Autodesk Fusion 360 part; units mm, degrees
(part 9 of 25)
  arc A995 (66.6606, 9.2438) -> (66.5391, 8.9505) centre (66.5999, 9.0972) ccw
  line L140 (79.2435, 6.4262) -> (79.2526, 6.4041)
  line L141 (68.5458, 9.1821) -> (70.8777, 6.8502)
  arc A996 (79.3901, 6.4869) -> (79.0968, 6.3655) centre (79.2435, 6.4262) ccw
  line L142 (75.7433, 6.4041) -> (75.7524, 6.4262)
  line L143 (82.2457, 6.4041) -> (82.5144, 7.053)
  arc A997 (74.5979, 9.0106) -> (74.5979, 9.3281) centre (74.5979, 9.1694) ccw
  line L144 (75.7524, 6.4262) -> (79.2435, 6.4262)
  line L145 (73.2468, 8.9006) -> (72.7502, 8.4041)
  arc A998 (73.8956, 9.3281) -> (73.8956, 9.0106) centre (73.8956, 9.1694) ccw
  line L146 (66.2472, 9.4498) -> (66.5998, 9.0972)
  arc A999 (66.4876, 8.9849) -> (66.7121, 9.2094) centre (66.5999, 9.0972) ccw
  line L147 (72.7411, 8.382) -> (72.1118, 8.382)
  arc A1000 (67.0606, 11.5724) -> (67.0606, 11.2549) centre (67.0606, 11.4137) ccw
  arc A1001 (75.631, 8.2918) -> (75.8555, 8.5163) centre (75.7433, 8.4041) ccw
  line L148 (66.2472, 10.8702) -> (66.0563, 10.4094)
  line L149 (72.1118, 8.382) -> (69.5048, 10.989)
  arc A1002 (67.5594, 11.2549) -> (67.5594, 11.5724) centre (67.5594, 11.4137) ccw
  arc A1003 (79.8099, 6.0542) -> (79.6884, 5.7609) centre (79.7492, 5.9076) ccw
  arc A1004 (72.6379, 8.5163) -> (72.8624, 8.2918) centre (72.7501, 8.4041) ccw
  line L150 (81.7491, 5.9076) -> (82.2457, 6.4041)
  arc A1005 (71.0405, 6.4628) -> (71.2651, 6.6873) centre (71.1528, 6.5751) ccw
  line L151 (79.7492, 5.9076) -> (80.398, 5.6388)
  arc A1006 (72.6035, 6.3434) -> (72.8969, 6.4649) centre (72.7502, 6.4042) ccw
  arc A1007 (81.1003, 5.4801) -> (81.1003, 5.7976) centre (81.1003, 5.6389) ccw
  arc A1008 (70.99, 6.9624) -> (70.7655, 6.7379) centre (70.8778, 6.8501) ccw
  arc A1009 (68.5458, 9.0234) -> (68.5458, 9.3408) centre (68.5458, 9.1821) ccw
  arc A1010 (75.8555, 6.2919) -> (75.631, 6.5164) centre (75.7433, 6.4041) ccw
  arc A1011 (67.4986, 9.053) -> (67.6201, 8.7596) centre (67.5593, 8.9063) ccw
  line L152 (80.398, 5.6388) -> (81.1003, 5.6388)
  line L153 (70.8777, 6.8502) -> (71.1528, 6.5751)
  arc A1012 (79.6369, 5.7953) -> (79.8614, 6.0198) centre (79.7491, 5.9076) ccw
  arc A1013 (71.2136, 6.7217) -> (71.0921, 6.4284) centre (71.1529, 6.5751) ccw
  line L154 (68.1051, 9.1821) -> (68.5458, 9.1821)
  line L155 (68.0202, 9.0972) -> (68.1051, 9.1821)
  line L156 (72.7411, 6.4262) -> (72.7502, 6.4041)
  line L157 (81.1003, 5.6388) -> (81.7491, 5.9076)
  line L158 (71.1528, 6.5751) -> (71.5122, 6.4262)
  arc A1014 (81.0395, 5.7855) -> (81.161, 5.4921) centre (81.1003, 5.6388) ccw
  line L159 (1.1279, 35.1317) -> (0.9017, 34.5856)
  arc A1015 (74.5371, 5.7855) -> (74.6586, 5.4921) centre (74.5978, 5.6388) ccw
  arc A1016 (60.0182, 19.5923) -> (59.7936, 19.8168) centre (59.9059, 19.7046) ccw
  arc A1017 (59.7936, 20.8232) -> (60.0182, 21.0477) centre (59.9059, 20.9355) ccw
  line L160 (0.9017, 34.5856) -> (0.9017, 33.9944)
  arc A1018 (1.0605, 34.5856) -> (0.7429, 34.5856) centre (0.9017, 34.5856) ccw
  line L161 (0.9017, 33.9944) -> (1.1279, 33.4483)
  arc A1019 (68.658, 9.2944) -> (68.4335, 9.0698) centre (68.5457, 9.1821) ccw
  line L162 (74.5979, 5.6388) -> (75.2467, 5.9076)
  arc A1020 (72.8624, 6.5164) -> (72.6379, 6.2919) centre (72.7501, 6.4041) ccw
  arc A1021 (68.0809, 8.9505) -> (67.9594, 9.2438) centre (68.0202, 9.0972) ccw
  arc A1022 (73.1345, 5.7953) -> (73.359, 6.0198) centre (73.2468, 5.9076) ccw
  arc A1023 (72.8877, 6.4869) -> (72.5944, 6.3655) centre (72.7411, 6.4262) ccw
  arc A1024 (68.2174, 9.0698) -> (67.9928, 9.2944) centre (68.1051, 9.1821) ccw
  line L163 (73.2468, 5.9076) -> (73.8956, 5.6388)
  arc A1025 (70.7655, 6.7379) -> (70.99, 6.9624) centre (70.8778, 6.8502) ccw
  line L164 (75.2467, 5.9076) -> (75.7433, 6.4041)
  arc A1026 (75.8991, 6.3655) -> (75.6058, 6.4869) centre (75.7525, 6.4262) ccw
  arc A1027 (82.3579, 6.2919) -> (82.1334, 6.5164) centre (82.2456, 6.4041) ccw
  line L165 (79.2526, 6.4041) -> (79.7492, 5.9076)
  arc A1028 (79.3648, 6.5164) -> (79.1403, 6.2919) centre (79.2525, 6.4042) ccw
  arc A1029 (71.5122, 6.585) -> (71.5122, 6.2675) centre (71.5122, 6.4263) ccw
  arc A1030 (80.398, 5.7976) -> (80.398, 5.4801) centre (80.398, 5.6389) ccw
  arc A1031 (81.8099, 5.7609) -> (81.6883, 6.0542) centre (81.7491, 5.9076) ccw
  line L166 (72.7502, 6.4041) -> (73.2468, 5.9076)
  arc A1032 (83.8136, 11.3225) -> (83.4961, 11.3225) centre (83.6548, 11.3225) ccw
  line L167 (73.8956, 5.6388) -> (74.5979, 5.6388)
  arc A1033 (75.5966, 6.4649) -> (75.89, 6.3434) centre (75.7433, 6.4041) ccw
  arc A1034 (73.8348, 5.4921) -> (73.9563, 5.7855) centre (73.8956, 5.6388) ccw
  arc A1035 (1.2746, 35.0709) -> (0.9812, 35.1924) centre (1.1279, 35.1316) ccw
  line L168 (71.5122, 6.4262) -> (72.7411, 6.4262)
  line L169 (82.5144, 7.053) -> (82.5144, 7.7552)
  arc A1036 (75.7524, 6.585) -> (75.7524, 6.2675) centre (75.7524, 6.4263) ccw
  arc A1037 (73.3075, 6.0542) -> (73.186, 5.7609) centre (73.2468, 5.9076) ccw
  arc A1038 (0.7429, 33.9944) -> (1.0605, 33.9944) centre (0.9017, 33.9944) ccw
  arc A1039 (82.6611, 6.9922) -> (82.3678, 7.1137) centre (82.5145, 7.053) ccw
  arc A1040 (71.4515, 6.2795) -> (71.573, 6.5729) centre (71.5122, 6.4262) ccw
  arc A1041 (73.8956, 5.7976) -> (73.8956, 5.4801) centre (73.8956, 5.6389) ccw
  arc A1042 (75.1344, 6.0198) -> (75.359, 5.7953) centre (75.2467, 5.9075) ccw
  arc A1043 (79.1059, 6.3434) -> (79.3993, 6.4649) centre (79.2526, 6.4041) ccw
  arc A1044 (68.1051, 9.3408) -> (68.1051, 9.0234) centre (68.1051, 9.1821) ccw
  arc A1045 (6.6867, 33.177) -> (6.5652, 32.8836) centre (6.626, 33.0303) ccw
  arc A1046 (84.2752, 11.7183) -> (84.0506, 11.9428) centre (84.1629, 11.8305) ccw
  arc A1047 (57.0464, 19.8168) -> (56.8218, 19.5923) centre (56.9341, 19.7046) ccw
  arc A1048 (57.6923, 18.7218) -> (57.9168, 18.9464) centre (57.8045, 18.8341) ccw
  line L170 (83.2309, 8.5029) -> (83.506, 8.778)
  arc A1049 (82.652, 7.8381) -> (82.3586, 7.7165) centre (82.5053, 7.7773) ccw
  arc A1050 (60.0646, 20.9355) -> (59.7471, 20.9355) centre (59.9059, 20.9355) ccw
  line L171 (57.8045, 21.8059) -> (56.9341, 20.9355)
  line L172 (4.004, 35.7759) -> (2.092, 35.7759)
  line L173 (82.5053, 7.7773) -> (83.2309, 8.5029)
  arc A1051 (59.1477, 21.9182) -> (58.9232, 21.6936) centre (59.0355, 21.8059) ccw
  arc A1052 (1.0484, 34.0552) -> (0.755, 33.9337) centre (0.9017, 33.9945) ccw
  arc A1053 (82.3557, 7.053) -> (82.6732, 7.053) centre (82.5145, 7.053) ccw
  line L174 (83.506, 8.778) -> (83.6549, 9.1374)
  arc A1054 (57.8045, 21.9646) -> (57.8045, 21.6471) centre (57.8045, 21.8059) ccw
  arc A1055 (83.3432, 8.3907) -> (83.1187, 8.6152) centre (83.231, 8.5029) ccw
  arc A1056 (59.0355, 18.6753) -> (59.0355, 18.9929) centre (59.0355, 18.8341) ccw
  arc A1057 (57.0928, 20.9355) -> (56.7754, 20.9355) centre (56.9341, 20.9355) ccw
  line L175 (82.5144, 7.7552) -> (82.5053, 7.7773)
  arc A1058 (1.6582, 35.4374) -> (1.4336, 35.6619) centre (1.5459, 35.5496) ccw
  arc A1059 (2.092, 35.9346) -> (2.092, 35.6171) centre (2.092, 35.7759) ccw
  arc A1060 (1.0157, 35.2439) -> (1.2402, 35.0194) centre (1.1279, 35.1317) ccw
  arc A1061 (0.9812, 33.3876) -> (1.2746, 33.5091) centre (1.1279, 33.4484) ccw
  arc A1062 (83.3594, 8.8388) -> (83.6527, 8.7173) centre (83.5061, 8.7781) ccw
  line L176 (59.0355, 18.8341) -> (59.9059, 19.7045)
  arc A1063 (0.755, 34.6463) -> (1.0484, 34.5248) centre (0.9017, 34.5855) ccw
  arc A1064 (83.5426, 11.4348) -> (83.7672, 11.2103) centre (83.6549, 11.3225) ccw
  line L177 (83.6549, 9.1374) -> (83.6549, 11.3225)
  arc A1065 (83.4961, 9.1374) -> (83.8136, 9.1374) centre (83.6548, 9.1374) ccw
  arc A1066 (57.8045, 18.9929) -> (57.8045, 18.6753) centre (57.8045, 18.8341) ccw
  arc A1067 (82.099, 6.4649) -> (82.3924, 6.3434) centre (82.2457, 6.4042) ccw
  arc A1068 (82.393, 7.8896) -> (82.6175, 7.665) centre (82.5053, 7.7773) ccw
  arc A1069 (4.004, 35.6171) -> (4.004, 35.9346) centre (4.004, 35.7759) ccw
  arc A1070 (1.4852, 35.6963) -> (1.6067, 35.403) centre (1.5459, 35.5496) ccw
  arc A1071 (83.1187, 8.6152) -> (83.3432, 8.3907) centre (83.231, 8.503) ccw
  line L178 (2.092, 35.7759) -> (1.5459, 35.5497)
  arc A1072 (58.9232, 18.9464) -> (59.1477, 18.7218) centre (59.0355, 18.8341) ccw
  arc A1073 (82.3678, 7.6945) -> (82.6611, 7.816) centre (82.5145, 7.7553) ccw
  line L179 (59.9059, 19.7045) -> (59.9059, 20.9355)
  line L180 (59.0355, 21.8059) -> (57.8045, 21.8059)
  line L181 (56.9341, 20.9355) -> (56.9341, 19.7045)
  arc A1074 (2.1528, 35.6292) -> (2.0313, 35.9226) centre (2.092, 35.7759) ccw
  arc A1075 (57.9168, 21.6936) -> (57.6923, 21.9182) centre (57.8046, 21.8059) ccw
  arc A1076 (56.8218, 21.0477) -> (57.0464, 20.8232) centre (56.9341, 20.9354) ccw
  line L182 (56.9341, 19.7045) -> (57.8045, 18.8341)
  line L183 (1.5459, 35.5497) -> (1.1279, 35.1317)
  line L184 (59.9059, 20.9355) -> (59.0355, 21.8059)
  arc A1077 (17.4808, 44.6377) -> (17.7053, 44.8622) centre (17.593, 44.7499) ccw
  arc A1078 (56.7754, 19.7045) -> (57.0928, 19.7045) centre (56.9341, 19.7045) ccw
  arc A1079 (83.6183, 8.6658) -> (83.3938, 8.8903) centre (83.5061, 8.7781) ccw
  arc A1080 (83.8016, 9.0767) -> (83.5082, 9.1982) centre (83.6549, 9.1374) ccw
  arc A1081 (59.0355, 21.6471) -> (59.0355, 21.9646) centre (59.0355, 21.8059) ccw
  arc A1082 (59.7471, 19.7045) -> (60.0646, 19.7045) centre (59.9059, 19.7045) ccw
  arc A1083 (17.8886, 31.7487) -> (17.5952, 31.8702) centre (17.7419, 31.8095) ccw
  line L185 (4.5501, 33.0303) -> (4.8319, 33.3121)
  arc A1084 (82.6732, 7.7552) -> (82.3557, 7.7552) centre (82.5145, 7.7552) ccw
  arc A1085 (3.9432, 32.9508) -> (4.0647, 32.6574) centre (4.004, 32.8041) ccw
  line L186 (83.6549, 11.3225) -> (84.1629, 11.8305)
  line L187 (57.8045, 18.8341) -> (59.0355, 18.8341)
  line L188 (2.092, 32.8041) -> (4.004, 32.8041)
  arc A1086 (12.5878, 29.7976) -> (12.4663, 29.5043) centre (12.5271, 29.651) ccw
  arc A1087 (4.4378, 33.1426) -> (4.6623, 32.9181) centre (4.55, 33.0304) ccw
  arc A1088 (15.8547, 29.5043) -> (15.7332, 29.7976) centre (15.7939, 29.651) ccw
  arc A1089 (15.3738, 29.6488) -> (15.4953, 29.3554) centre (15.4345, 29.5021) ccw
  arc A1090 (4.6108, 32.8836) -> (4.4893, 33.177) centre (4.5501, 33.0303) ccw
  line L189 (17.593, 31.4501) -> (17.7419, 31.8095)
  arc A1091 (9.0232, 32.9508) -> (9.1447, 32.6574) centre (9.084, 32.8041) ccw
  arc A1092 (15.6817, 29.7632) -> (15.9062, 29.5387) centre (15.794, 29.651) ccw
  line L190 (12.8865, 29.5021) -> (15.4345, 29.5021)
  arc A1093 (9.084, 32.6454) -> (9.084, 32.9628) centre (9.084, 32.8041) ccw
  line L191 (12.5271, 29.651) -> (12.8865, 29.5021)
  arc A1094 (17.5831, 31.8095) -> (17.9006, 31.8095) centre (17.7419, 31.8095) ccw
  arc A1095 (17.4464, 31.5108) -> (17.7397, 31.3893) centre (17.5931, 31.4501) ccw
  line L192 (17.3179, 45.025) -> (15.1096, 47.2333)
  arc A1096 (6.3441, 33.1534) -> (6.3441, 33.4708) centre (6.3441, 33.3121) ccw
  arc A1097 (9.3498, 32.7424) -> (9.2283, 33.0357) centre (9.2891, 32.8891) ccw
  line L193 (1.1279, 33.4483) -> (1.5459, 33.0303)
  arc A1098 (6.5136, 32.9181) -> (6.7382, 33.1426) centre (6.6259, 33.0304) ccw
  arc A1099 (15.2219, 47.3456) -> (14.9974, 47.1211) centre (15.1097, 47.2334) ccw
  line L194 (15.1096, 47.2333) -> (15.24, 47.3637)
  arc A1100 (17.7397, 44.8107) -> (17.4464, 44.6892) centre (17.5931, 44.7499) ccw
  line L195 (17.593, 44.7499) -> (17.3179, 45.025)
  arc A1101 (19.9142, 47.1562) -> (19.77, 47.4391) centre (19.8421, 47.2977) ccw
  arc A1102 (17.4302, 45.1373) -> (17.2057, 44.9128) centre (17.318, 45.025) ccw
  line L196 (1.5459, 33.0303) -> (2.092, 32.8041)
  arc A1103 (20.1279, 47.309) -> (19.9412, 47.5659) centre (20.0346, 47.4375) ccw
  line L197 (17.7419, 31.8095) -> (17.7419, 44.3905)
  arc A1104 (1.6067, 33.177) -> (1.4852, 32.8836) centre (1.546, 33.0303) ccw
  arc A1105 (4.004, 32.6454) -> (4.004, 32.9628) centre (4.004, 32.8041) ccw
  line L198 (9.084, 32.8041) -> (9.289, 32.889)
  arc A1106 (7.172, 32.9628) -> (7.172, 32.6454) centre (7.172, 32.8041) ccw
  arc A1107 (4.9441, 33.1998) -> (4.7196, 33.4244) centre (4.8319, 33.3121) ccw
  line L199 (4.8319, 33.3121) -> (6.3441, 33.3121)
  arc A1108 (17.2057, 44.9128) -> (17.4302, 45.1373) centre (17.3179, 45.0251) ccw
  arc A1109 (1.2402, 33.5606) -> (1.0157, 33.336) centre (1.128, 33.4483) ccw
  arc A1110 (15.3523, 47.2514) -> (15.1277, 47.4759) centre (15.24, 47.3636) ccw
  arc A1111 (12.8257, 29.3554) -> (12.9472, 29.6488) centre (12.8865, 29.5021) ccw
  line L200 (17.7419, 44.3905) -> (17.593, 44.7499)
  line L201 (6.3441, 33.3121) -> (6.6259, 33.0303)
  arc A1112 (12.8865, 29.6609) -> (12.8865, 29.3434) centre (12.8865, 29.5022) ccw
  line L202 (15.24, 47.3637) -> (15.51, 47.0937)
  arc A1113 (9.4013, 33.0013) -> (9.1768, 32.7768) centre (9.2891, 32.8891) ccw
  line L203 (7.172, 32.8041) -> (9.084, 32.8041)
  arc A1114 (7.1113, 32.6574) -> (7.2328, 32.9508) centre (7.1721, 32.8041) ccw
  arc A1115 (15.4345, 29.3434) -> (15.4345, 29.6609) centre (15.4345, 29.5022) ccw
  arc A1116 (6.4564, 33.4244) -> (6.2319, 33.1998) centre (6.3442, 33.3121) ccw
  arc A1117 (1.4336, 32.9181) -> (1.6582, 33.1426) centre (1.5459, 33.0304) ccw
  arc A1118 (12.4148, 29.5387) -> (12.6393, 29.7632) centre (12.5271, 29.651) ccw
  arc A1119 (17.7053, 31.3378) -> (17.4808, 31.5623) centre (17.593, 31.4501) ccw
  line L204 (15.4345, 29.5021) -> (15.7939, 29.651)
  line L205 (4.004, 32.8041) -> (4.5501, 33.0303)
  line L206 (6.6259, 33.0303) -> (7.172, 32.8041)
  arc A1120 (2.0313, 32.6574) -> (2.1528, 32.9508) centre (2.0921, 32.8041) ccw
  arc A1121 (4.8319, 33.4708) -> (4.8319, 33.1534) centre (4.8319, 33.3121) ccw
  arc A1122 (2.092, 32.9628) -> (2.092, 32.6454) centre (2.092, 32.8041) ccw
  line L207 (15.7939, 29.651) -> (17.593, 31.4501)
  arc A1123 (17.9006, 44.3905) -> (17.5831, 44.3905) centre (17.7419, 44.3905) ccw
  arc A1124 (17.5952, 44.3298) -> (17.8886, 44.4513) centre (17.7419, 44.3905) ccw
  arc A1125 (14.9974, 47.3456) -> (15.2219, 47.1211) centre (15.1097, 47.2334) ccw
  line L208 (9.289, 32.889) -> (12.5271, 29.651)
  arc A1126 (20.2526, 47.431) -> (20.0281, 47.6555) centre (20.1403, 47.5433) ccw
  arc A1127 (21.1781, 46.6782) -> (21.2996, 46.9716) centre (21.2388, 46.8249) ccw
  line L209 (19.4039, 47.1161) -> (19.6301, 47.1896)
  arc A1128 (16.8611, 46.6662) -> (16.8611, 46.9836) centre (16.8611, 46.8249) ccw
  arc A1129 (18.0719, 47.6555) -> (17.8473, 47.431) centre (17.9596, 47.5433) ccw
  arc A1130 (18.9062, 46.9221) -> (18.9559, 47.2357) centre (18.9311, 47.0789) ccw
  arc A1131 (19.05, 49.3712) -> (19.05, 49.6887) centre (19.05, 49.53) ccw
  arc A1132 (19.2088, 49.53) -> (18.8913, 49.53) centre (19.0501, 49.53) ccw
  line L210 (20.1404, 47.5433) -> (20.59, 47.0937)
  line L211 (19.05, 47.0789) -> (19.05, 49.53)
  line L212 (16.1589, 46.8249) -> (16.8611, 46.8249)
  line L213 (19.05, 49.53) -> (19.05, 47.0789)
  arc A1133 (18.5189, 47.3406) -> (18.4208, 47.0386) centre (18.4699, 47.1896) ccw
  arc A1134 (18.33, 47.4391) -> (18.1858, 47.1562) centre (18.2579, 47.2977) ccw
  arc A1135 (19.5581, 47.3311) -> (19.7022, 47.0482) centre (19.6302, 47.1897) ccw
  line L214 (18.2579, 47.2976) -> (18.4699, 47.1896)
  arc A1136 (17.9532, 47.3252) -> (18.1777, 47.5497) centre (18.0655, 47.4375) ccw
  line L215 (19.05, 47.0789) -> (19.1689, 47.0789)
  line L216 (17.9596, 47.5433) -> (18.0655, 47.4374)
  line L217 (17.51, 47.0937) -> (17.9596, 47.5433)
  line L218 (15.51, 47.0937) -> (16.1589, 46.8249)
  arc A1137 (19.1441, 47.2357) -> (19.1938, 46.9221) centre (19.169, 47.0789) ccw
  arc A1138 (17.3977, 47.2059) -> (17.6222, 46.9814) centre (17.5099, 47.0936) ccw
  arc A1139 (19.7488, 47.426) -> (19.9354, 47.1692) centre (19.8421, 47.2976) ccw
  line L219 (20.0345, 47.4374) -> (20.1404, 47.5433)
  line L220 (19.6301, 47.1896) -> (19.8421, 47.2976)
  arc A1140 (16.1589, 46.9836) -> (16.1589, 46.6662) centre (16.1589, 46.8249) ccw
  line L221 (18.4699, 47.1896) -> (18.6961, 47.1161)
  arc A1141 (15.3523, 47.4759) -> (15.1277, 47.2514) centre (15.24, 47.3636) ccw
  line L222 (18.6961, 47.1161) -> (18.9311, 47.0789)
  arc A1142 (18.7209, 47.2729) -> (18.6713, 46.9593) centre (18.6961, 47.1161) ccw
  line L223 (19.8421, 47.2976) -> (20.0345, 47.4374)
  line L224 (18.9311, 47.0789) -> (19.05, 47.0789)
  arc A1143 (19.1689, 46.9202) -> (19.1689, 47.2377) centre (19.1689, 47.0789) ccw
  arc A1144 (18.8912, 47.0789) -> (19.2087, 47.0789) centre (19.05, 47.0789) ccw
  arc A1145 (19.6792, 47.0386) -> (19.5811, 47.3406) centre (19.6302, 47.1896) ccw
  line L225 (20.59, 47.0937) -> (21.2389, 46.8249)
  arc A1146 (18.1646, 47.1692) -> (18.3512, 47.426) centre (18.2579, 47.2976) ccw
  arc A1147 (18.3978, 47.0482) -> (18.5419, 47.3311) centre (18.4699, 47.1897) ccw
  arc A1148 (15.5708, 47.2403) -> (15.4493, 46.947) centre (15.51, 47.0936) ccw
  line L226 (16.8611, 46.8249) -> (17.51, 47.0937)
  arc A1149 (19.4287, 46.9593) -> (19.3791, 47.2729) centre (19.4039, 47.1161) ccw
  arc A1150 (18.8913, 47.0789) -> (19.2088, 47.0789) centre (19.0501, 47.0789) ccw
  arc A1151 (19.05, 49.6887) -> (19.05, 49.3712) centre (19.05, 49.53) ccw
  arc A1152 (19.05, 47.2377) -> (19.05, 46.9202) centre (19.05, 47.0789) ccw
  line L227 (18.0655, 47.4374) -> (18.2579, 47.2976)
  line L228 (19.1689, 47.0789) -> (19.4039, 47.1161)
  arc A1153 (17.5707, 46.947) -> (17.4492, 47.2403) centre (17.5099, 47.0936) ccw
  arc A1154 (19.05, 46.9202) -> (19.05, 47.2377) centre (19.05, 47.0789) ccw
  arc A1155 (16.8004, 46.9716) -> (16.9219, 46.6782) centre (16.8611, 46.8249) ccw
  arc A1156 (19.9223, 47.5497) -> (20.1468, 47.3252) centre (20.0346, 47.4375) ccw
  arc A1157 (15.3978, 46.9814) -> (15.6223, 47.2059) centre (15.51, 47.0936) ccw
  arc A1158 (18.0719, 47.431) -> (17.8473, 47.6555) centre (17.9596, 47.5433) ccw
  arc A1159 (19.3548, 47.2671) -> (19.453, 46.9651) centre (19.4039, 47.1161) ccw
  arc A1160 (18.1588, 47.5659) -> (17.9721, 47.309) centre (18.0654, 47.4375) ccw
  arc A1161 (20.2526, 47.6555) -> (20.0281, 47.431) centre (20.1403, 47.5433) ccw
  arc A1162 (20.4778, 46.9814) -> (20.7023, 47.2059) centre (20.59, 47.0936) ccw
  arc A1163 (20.6508, 47.2403) -> (20.5293, 46.947) centre (20.59, 47.0936) ccw
  arc A1164 (18.9311, 47.2377) -> (18.9311, 46.9202) centre (18.9311, 47.0789) ccw
  arc A1165 (16.0981, 46.6782) -> (16.2196, 46.9716) centre (16.1589, 46.8249) ccw
  arc A1166 (18.647, 46.9651) -> (18.7452, 47.2671) centre (18.6961, 47.1161) ccw
  arc A1167 (27.0488, 48.5057) -> (26.8621, 48.2488) centre (26.9554, 48.3773) ccw
  arc A1168 (25.6904, 47.9114) -> (25.8119, 47.618) centre (25.7511, 47.7647) ccw
  arc A1169 (22.6507, 46.947) -> (22.5292, 47.2403) centre (22.59, 47.0936) ccw
  line L229 (24.4, 48.0335) -> (25.0489, 47.7647)
  arc A1170 (21.8804, 46.9716) -> (22.0019, 46.6782) centre (21.9411, 46.8249) ccw
  arc A1171 (27.7962, 47.8619) -> (27.8459, 48.1755) centre (27.8211, 48.0187) ccw
  arc A1172 (24.9881, 47.618) -> (25.1096, 47.9114) centre (25.0489, 47.7647) ccw
  arc A1173 (24.1587, 48.4993) -> (23.9342, 48.2747) centre (24.0465, 48.387) ccw
  arc A1174 (28.3187, 47.8991) -> (28.2691, 48.2127) centre (28.2939, 48.0559) ccw
  arc A1175 (23.1965, 48.2391) -> (23.514, 48.2391) centre (23.3553, 48.2391) ccw
  arc A1176 (28.0589, 47.86) -> (28.0589, 48.1775) centre (28.0589, 48.0187) ccw
  arc A1177 (27.8211, 48.1774) -> (27.8211, 47.86) centre (27.8211, 48.0187) ccw
  arc A1178 (25.7511, 47.606) -> (25.7511, 47.9235) centre (25.7511, 47.7648) ccw
  arc A1179 (26.9619, 48.5953) -> (26.7373, 48.3708) centre (26.8496, 48.4831) ccw
  arc A1180 (26.4607, 47.8868) -> (26.3392, 48.1801) centre (26.3999, 48.0335) ccw
  arc A1181 (24.2878, 47.9212) -> (24.5123, 48.1457) centre (24.4001, 48.0335) ccw
  arc A1182 (27.0546, 48.109) -> (27.2412, 48.3658) centre (27.1479, 48.2374) ccw
  arc A1183 (23.1988, 47.478) -> (22.9743, 47.7025) centre (23.0866, 47.5903) ccw
  line L230 (26.4, 48.0335) -> (26.8496, 48.4831)
  line L231 (27.1479, 48.2374) -> (27.3599, 48.1294)
  arc A1184 (27.22, 48.3789) -> (27.0758, 48.096) centre (27.1479, 48.2374) ccw
  arc A1185 (27.94, 48.1775) -> (27.94, 47.86) centre (27.94, 48.0187) ccw
  arc A1186 (21.2389, 46.9836) -> (21.2389, 46.6662) centre (21.2389, 46.8249) ccw
  line L232 (27.3599, 48.1294) -> (27.5861, 48.0559)
  line L233 (25.7511, 47.7647) -> (26.4, 48.0335)
  line L234 (21.2389, 46.8249) -> (21.9411, 46.8249)
  arc A1187 (23.502, 48.1783) -> (23.2086, 48.2998) centre (23.3553, 48.239) ccw
  line L235 (23.3553, 48.387) -> (24.0465, 48.387)
  arc A1188 (27.537, 47.9049) -> (27.6352, 48.2069) centre (27.5861, 48.0559) ccw
  arc A1189 (26.9619, 48.3708) -> (26.7373, 48.5953) centre (26.8496, 48.483) ccw
  arc A1190 (28.0987, 49.53) -> (27.7812, 49.53) centre (27.94, 49.53) ccw
  line L236 (21.9411, 46.8249) -> (22.59, 47.0937)
  arc A1191 (26.2877, 48.1457) -> (26.5122, 47.9212) centre (26.4, 48.0335) ccw
  arc A1192 (27.2878, 47.988) -> (27.4319, 48.2709) centre (27.3599, 48.1294) ccw
  arc A1193 (19.2087, 49.53) -> (18.8912, 49.53) centre (19.05, 49.53) ccw
  arc A1194 (28.0988, 49.53) -> (27.7813, 49.53) centre (27.9401, 49.53) ccw
  arc A1195 (26.8432, 48.265) -> (27.0677, 48.4895) centre (26.9554, 48.3773) ccw
  line L237 (23.0865, 47.5902) -> (23.3553, 48.2391)
  arc A1196 (27.4089, 48.2804) -> (27.3108, 47.9784) centre (27.3599, 48.1294) ccw
  arc A1197 (21.9411, 46.6662) -> (21.9411, 46.9836) centre (21.9411, 46.8249) ccw
  line L238 (27.8211, 48.0187) -> (27.94, 48.0187)
  arc A1198 (25.0489, 47.9235) -> (25.0489, 47.606) centre (25.0489, 47.7648) ccw
  arc A1199 (27.94, 47.8599) -> (27.94, 48.1774) centre (27.94, 48.0187) ccw
  line L239 (22.59, 47.0937) -> (23.0865, 47.5902)
  arc A1200 (24.4608, 48.1801) -> (24.3393, 47.8868) centre (24.4, 48.0335) ccw
  line L240 (27.5861, 48.0559) -> (27.8211, 48.0187)
  line L241 (27.94, 48.0187) -> (28.0589, 48.0187)
  line L242 (28.0589, 48.0187) -> (28.2939, 48.0559)
  line L243 (24.0465, 48.387) -> (24.4, 48.0335)
  arc A1201 (22.9399, 47.651) -> (23.2332, 47.5295) centre (23.0866, 47.5903) ccw
  arc A1202 (27.6109, 48.2127) -> (27.5613, 47.8991) centre (27.5861, 48.0559) ccw
  arc A1203 (27.7813, 48.0187) -> (28.0988, 48.0187) centre (27.9401, 48.0187) ccw
  arc A1204 (24.0465, 48.2283) -> (24.0465, 48.5457) centre (24.0465, 48.387) ccw
  arc A1205 (22.4777, 47.2059) -> (22.7022, 46.9814) centre (22.5899, 47.0936) ccw
  line L244 (25.0489, 47.7647) -> (25.7511, 47.7647)
  arc A1206 (27.94, 49.3712) -> (27.94, 49.6887) centre (27.94, 49.53) ccw
  arc A1207 (23.514, 48.387) -> (23.1965, 48.387) centre (23.3553, 48.387) ccw
  line L245 (26.9555, 48.3772) -> (27.1479, 48.2374)
  arc A1208 (23.3553, 48.5457) -> (23.3553, 48.2283) centre (23.3553, 48.387) ccw
  line L246 (23.3553, 48.2391) -> (23.3553, 48.387)
  line L247 (26.8496, 48.4831) -> (26.9555, 48.3772)
  line L248 (30.48, 49.53) -> (30.48, 48.0187)
  line L249 (30.8339, 48.0559) -> (31.0601, 48.1294)
  arc A1209 (28.6388, 48.3658) -> (28.8254, 48.109) centre (28.7321, 48.2374) ccw
  arc A1210 (30.48, 49.6887) -> (30.48, 49.3712) centre (30.48, 49.53) ccw
  line L250 (29.6879, 48.2374) -> (29.8999, 48.1294)
  arc A1211 (29.3384, 48.8001) -> (29.0816, 48.6135) centre (29.21, 48.7068) ccw
  line L251 (29.21, 48.7068) -> (29.3272, 48.5455)
  arc A1212 (29.3832, 48.265) -> (29.6077, 48.4895) centre (29.4955, 48.3773) ccw
  arc A1213 (29.3384, 48.6135) -> (29.0816, 48.8001) centre (29.21, 48.7068) ccw
  line L252 (29.0928, 48.5455) -> (29.21, 48.7068)
  arc A1214 (27.94, 49.6887) -> (27.94, 49.3712) centre (27.94, 49.53) ccw
  line L253 (31.0601, 48.1294) -> (31.2721, 48.2374)
  arc A1215 (28.2448, 48.2069) -> (28.343, 47.9049) centre (28.2939, 48.0559) ccw
  line L254 (31.2721, 48.2374) -> (31.4645, 48.3772)
  arc A1216 (31.3442, 48.096) -> (31.2, 48.3789) centre (31.2721, 48.2375) ccw
  arc A1217 (30.3212, 48.0187) -> (30.6387, 48.0187) centre (30.48, 48.0187) ccw
  arc A1218 (29.9489, 48.2804) -> (29.8508, 47.9784) centre (29.8999, 48.1294) ccw
  arc A1219 (28.8042, 48.096) -> (28.66, 48.3789) centre (28.7321, 48.2375) ccw
  arc A1220 (30.3213, 48.0187) -> (30.6388, 48.0187) centre (30.4801, 48.0187) ccw
  arc A1221 (29.8278, 47.988) -> (29.9719, 48.2709) centre (29.8999, 48.1294) ccw
  arc A1222 (30.3362, 47.8619) -> (30.3859, 48.1755) centre (30.3611, 48.0187) ccw
  line L255 (30.5989, 48.0187) -> (30.8339, 48.0559)
  arc A1223 (30.8587, 47.8991) -> (30.8091, 48.2127) centre (30.8339, 48.0559) ccw
  arc A1224 (28.5692, 47.9784) -> (28.4711, 48.2804) centre (28.5202, 48.1294) ccw
  arc A1225 (30.48, 47.8599) -> (30.48, 48.1774) centre (30.48, 48.0187) ccw
  line L256 (30.48, 48.0187) -> (30.5989, 48.0187)
  line L257 (28.9245, 48.3772) -> (29.0928, 48.5455)
  arc A1226 (30.3611, 48.1774) -> (30.3611, 47.86) centre (30.3611, 48.0187) ccw
  arc A1227 (29.0179, 48.2488) -> (28.8312, 48.5057) centre (28.9246, 48.3773) ccw
  arc A1228 (30.077, 47.9049) -> (30.1752, 48.2069) centre (30.1261, 48.0559) ccw
  arc A1229 (30.5741, 48.1755) -> (30.6238, 47.8619) centre (30.599, 48.0187) ccw
  line L258 (27.94, 48.0187) -> (27.94, 49.53)
  arc A1230 (28.8123, 48.4895) -> (29.0368, 48.265) centre (28.9246, 48.3773) ccw
  arc A1231 (28.4481, 48.2709) -> (28.5922, 47.988) centre (28.5202, 48.1294) ccw
  arc A1232 (30.1509, 48.2127) -> (30.1013, 47.8991) centre (30.1261, 48.0559) ccw
  arc A1233 (28.9643, 48.6388) -> (29.2212, 48.4521) centre (29.0928, 48.5455) ccw
  arc A1234 (29.5888, 48.5057) -> (29.4021, 48.2488) centre (29.4955, 48.3772) ccw
  line L259 (30.1261, 48.0559) -> (30.3611, 48.0187)
  line L260 (29.3272, 48.5455) -> (29.4955, 48.3772)
  line L261 (31.5704, 48.4831) -> (32.02, 48.0335)
  arc A1235 (30.5989, 47.86) -> (30.5989, 48.1775) centre (30.5989, 48.0187) ccw
  arc A1236 (30.48, 49.3712) -> (30.48, 49.6887) centre (30.48, 49.53) ccw
  line L262 (30.48, 48.0187) -> (30.48, 49.53)
  line L263 (28.2939, 48.0559) -> (28.5201, 48.1294)
  line L264 (31.4645, 48.3772) -> (31.5704, 48.4831)
  line L265 (29.4955, 48.3772) -> (29.6879, 48.2374)
  arc A1237 (31.3523, 48.4895) -> (31.5768, 48.265) centre (31.4645, 48.3773) ccw
  arc A1238 (29.205, 48.4332) -> (28.9805, 48.6577) centre (29.0927, 48.5455) ccw
  line L266 (28.7321, 48.2374) -> (28.9245, 48.3772)
  line L267 (30.3611, 48.0187) -> (30.48, 48.0187)
  arc A1239 (30.7848, 48.2069) -> (30.883, 47.9049) centre (30.8339, 48.0559) ccw
  arc A1240 (29.4395, 48.6577) -> (29.215, 48.4332) centre (29.3272, 48.5455) ccw
  line L268 (28.5201, 48.1294) -> (28.7321, 48.2374)
  arc A1241 (29.76, 48.3789) -> (29.6158, 48.096) centre (29.6879, 48.2374) ccw
  arc A1242 (29.1988, 48.4521) -> (29.4557, 48.6388) centre (29.3273, 48.5455) ccw
  line L269 (29.8999, 48.1294) -> (30.1261, 48.0559)
  arc A1243 (30.6388, 49.53) -> (30.3213, 49.53) centre (30.4801, 49.53) ccw
  arc A1244 (29.5946, 48.109) -> (29.7812, 48.3658) centre (29.6879, 48.2374) ccw
  line L270 (27.94, 49.53) -> (27.94, 48.0187)
  arc A1245 (31.1092, 47.9784) -> (31.0111, 48.2804) centre (31.0602, 48.1294) ccw
  arc A1246 (27.7812, 48.0187) -> (28.0987, 48.0187) centre (27.94, 48.0187) ccw
  line L271 (24.0548, 44.6572) -> (24.5156, 44.4663)
  arc A1247 (30.48, 48.1775) -> (30.48, 47.86) centre (30.48, 48.0187) ccw
  arc A1248 (34.5214, 47.8776) -> (34.6428, 48.171) centre (34.5821, 48.0243) ccw
  arc A1249 (25.5601, 46.8566) -> (25.5601, 46.5391) centre (25.5601, 46.6979) ccw
  arc A1250 (23.8144, 45.1221) -> (23.5899, 44.8976) centre (23.7021, 45.0099) ccw
  arc A1251 (25.4478, 46.5856) -> (25.6724, 46.8102) centre (25.5601, 46.6979) ccw
  line L272 (33.3711, 47.7647) -> (34.02, 48.0335)
  arc A1252 (28.0341, 48.1755) -> (28.0838, 47.8619) centre (28.059, 48.0187) ccw
  arc A1253 (32.6689, 47.9235) -> (32.6689, 47.606) centre (32.6689, 47.7648) ccw
  arc A1254 (33.8849, 46.5391) -> (33.8849, 46.8566) centre (33.8849, 46.6979) ccw
  line L273 (34.29, 48.3035) -> (34.56, 48.0335)
  arc A1255 (31.5579, 48.2488) -> (31.3712, 48.5057) centre (31.4646, 48.3773) ccw
  arc A1256 (34.4023, 48.1912) -> (34.1777, 48.4157) centre (34.29, 48.3035) ccw
  arc A1257 (24.5156, 44.6251) -> (24.5156, 44.3076) centre (24.5156, 44.4664) ccw
  line L274 (33.8849, 46.6979) -> (25.5601, 46.6979)
  arc A1258 (25.0144, 44.3076) -> (25.0144, 44.6251) centre (25.0144, 44.4664) ccw
  line L275 (25.0144, 44.4663) -> (25.4752, 44.6572)
  arc A1259 (23.658, 45.5314) -> (23.3646, 45.4099) centre (23.5113, 45.4706) ccw
  arc A1260 (24.4549, 44.3196) -> (24.5764, 44.613) centre (24.5157, 44.4663) ccw
  line L276 (34.56, 48.0335) -> (34.5821, 48.0243)
  arc A1261 (31.9078, 47.9212) -> (32.1323, 48.1457) centre (32.0201, 48.0335) ccw
  arc A1262 (34.7409, 48.0243) -> (34.4234, 48.0243) centre (34.5822, 48.0243) ccw
  arc A1263 (31.1788, 48.3658) -> (31.3654, 48.109) centre (31.2721, 48.2374) ccw
  line L277 (24.5156, 44.4663) -> (25.0144, 44.4663)
  line L278 (23.7022, 45.0098) -> (24.0548, 44.6572)
  arc A1264 (24.1156, 44.8038) -> (23.9941, 44.5105) centre (24.0549, 44.6572) ccw
  arc A1265 (33.3104, 47.9114) -> (33.4319, 47.618) centre (33.3711, 47.7647) ccw
  line L279 (34.5821, 47.3951) -> (33.8849, 46.6979)
  line L280 (23.7022, 46.4302) -> (23.5113, 45.9694)
  arc A1266 (25.0144, 46.8149) -> (25.0144, 47.1324) centre (25.0144, 46.9737) ccw
  arc A1267 (31.6826, 48.3708) -> (31.4581, 48.5953) centre (31.5704, 48.483) ccw
  arc A1268 (23.6701, 45.9694) -> (23.3526, 45.9694) centre (23.5113, 45.9694) ccw
  line L281 (23.5113, 45.9694) -> (23.5113, 45.4706)
  arc A1269 (33.3711, 47.606) -> (33.3711, 47.9235) centre (33.3711, 47.7648) ccw
  arc A1270 (34.4234, 47.3951) -> (34.7409, 47.3951) centre (34.5822, 47.3951) ccw
  arc A1271 (32.6081, 47.618) -> (32.7296, 47.9114) centre (32.6689, 47.7647) ccw
  arc A1272 (25.4144, 46.6362) -> (25.5359, 46.9295) centre (25.4752, 46.7828) ccw
  line L282 (32.02, 48.0335) -> (32.6689, 47.7647)
  arc A1273 (25.5359, 44.5105) -> (25.4144, 44.8038) centre (25.4752, 44.6572) ccw
  arc A1274 (24.1671, 46.6706) -> (23.9426, 46.8951) centre (24.0549, 46.7829) ccw
  arc A1275 (23.3646, 46.0301) -> (23.658, 45.9086) centre (23.5113, 45.9694) ccw
  line L283 (25.4752, 46.7828) -> (25.0144, 46.9737)
  arc A1276 (23.5555, 44.9491) -> (23.8488, 45.0706) centre (23.7021, 45.0099) ccw
  line L284 (32.6689, 47.7647) -> (33.3711, 47.7647)
  arc A1277 (34.4023, 48.4157) -> (34.1777, 48.1912) centre (34.29, 48.3035) ccw
  arc A1278 (30.9881, 48.2709) -> (31.1322, 47.988) centre (31.0602, 48.1294) ccw
  arc A1279 (30.6387, 49.53) -> (30.3212, 49.53) centre (30.48, 49.53) ccw
  arc A1280 (34.0807, 47.8868) -> (33.9592, 48.1801) centre (34.02, 48.0335) ccw
  arc A1281 (33.7727, 46.8102) -> (33.9972, 46.5856) centre (33.885, 46.6979) ccw
  line L285 (25.0144, 46.9737) -> (24.5156, 46.9737)
  arc A1282 (31.6826, 48.5953) -> (31.4581, 48.3708) centre (31.5704, 48.483) ccw
  line L286 (25.5601, 46.6979) -> (25.4752, 46.7828)
  arc A1283 (33.9077, 48.1457) -> (34.1322, 47.9212) centre (34.02, 48.0335) ccw
  line L287 (24.5156, 46.9737) -> (24.0548, 46.7828)
  line L288 (34.5821, 48.0243) -> (34.5821, 47.3951)
  arc A1284 (23.8488, 46.3694) -> (23.5555, 46.4909) centre (23.7021, 46.4301) ccw
  arc A1285 (34.6208, 48.1801) -> (34.4993, 47.8868) centre (34.56, 48.0335) ccw
  arc A1286 (34.6944, 47.2828) -> (34.4698, 47.5073) centre (34.5821, 47.395) ccw
  arc A1287 (25.5874, 46.8951) -> (25.3629, 46.6706) centre (25.4752, 46.7829) ccw
  arc A1288 (23.9941, 46.9295) -> (24.1156, 46.6362) centre (24.0549, 46.7828) ccw
  arc A1289 (24.9536, 44.613) -> (25.0751, 44.3196) centre (25.0144, 44.4663) ccw
  arc A1290 (24.5156, 47.1324) -> (24.5156, 46.8149) centre (24.5156, 46.9737) ccw
  arc A1291 (29.7976, 42.4032) -> (29.5043, 42.5247) centre (29.651, 42.4639) ccw
  line L289 (35.9156, 33.6167) -> (35.9156, 34.9633)
  arc A1292 (35.7568, 33.6167) -> (36.0743, 33.6167) centre (35.9156, 33.6167) ccw
  arc A1293 (24.5764, 46.827) -> (24.4549, 47.1204) centre (24.5156, 46.9737) ccw
  arc A1294 (29.3554, 42.1653) -> (29.6488, 42.0438) centre (29.5021, 42.1045) ccw
  line L290 (34.02, 48.0335) -> (34.29, 48.3035)
  arc A1295 (32.8567, 35.3802) -> (33.0812, 35.1556) centre (32.9689, 35.2679) ccw
  line L291 (31.5555, 33.3121) -> (32.969, 33.3121)
  arc A1296 (35.8033, 34.8511) -> (36.0279, 35.0756) centre (35.9156, 34.9634) ccw
  line L292 (23.5113, 45.4706) -> (23.7022, 45.0098)
  arc A1297 (31.0838, 33.3487) -> (31.3083, 33.5732) centre (31.196, 33.4609) ccw
  line L293 (29.9261, 42.739) -> (29.651, 42.4639)
  arc A1298 (29.3434, 35.3655) -> (29.6609, 35.3655) centre (29.5022, 35.3655) ccw
  arc A1299 (23.5899, 46.5424) -> (23.8144, 46.3179) centre (23.7021, 46.4301) ccw
  line L294 (34.9633, 35.9156) -> (33.6167, 35.9156)
  arc A1300 (34.9633, 35.7568) -> (34.9633, 36.0743) centre (34.9633, 35.9156) ccw
  arc A1301 (25.5601, 44.9008) -> (25.5601, 44.5834) centre (25.5601, 44.7421) ccw
  line L295 (29.5021, 42.1045) -> (29.5021, 35.3655)
  arc A1302 (29.9261, 34.8897) -> (29.9261, 34.5722) centre (29.9261, 34.7309) ccw
  line L296 (29.651, 42.4639) -> (29.5021, 42.1045)
  arc A1303 (30.8087, 33.6238) -> (31.0332, 33.8483) centre (30.921, 33.7361) ccw
  arc A1304 (30.0383, 42.6268) -> (29.8138, 42.8513) centre (29.9261, 42.7391) ccw
  arc A1305 (25.3629, 44.7694) -> (25.5874, 44.5449) centre (25.4751, 44.6571) ccw
  arc A1306 (23.9426, 44.5449) -> (24.1671, 44.7694) centre (24.0548, 44.6571) ccw
  line L297 (35.9156, 34.9633) -> (34.9633, 35.9156)
  line L298 (30.921, 33.7361) -> (31.1961, 33.461)
  arc A1307 (30.0383, 34.8432) -> (29.8138, 34.6187) centre (29.9261, 34.7309) ccw
  arc A1308 (31.4947, 33.1654) -> (31.6162, 33.4588) centre (31.5555, 33.3121) ccw
  arc A1309 (33.0812, 33.4244) -> (32.8567, 33.1998) centre (32.9689, 33.3121) ccw
  arc A1310 (36.0279, 33.5044) -> (35.8033, 33.7289) centre (35.9156, 33.6167) ccw
  arc A1311 (36.0743, 34.9633) -> (35.7568, 34.9633) centre (35.9156, 34.9633) ccw
  arc A1312 (34.8511, 32.7767) -> (35.0756, 32.5521) centre (34.9634, 32.6644) ccw
  arc A1313 (32.0414, 44.6298) -> (31.8169, 44.8544) centre (31.9292, 44.7421) ccw
  line L299 (29.651, 35.0061) -> (29.9261, 34.731)
  arc A1314 (29.8138, 34.6187) -> (30.0383, 34.8432) centre (29.9261, 34.7309) ccw
  arc A1315 (32.1551, 35.4266) -> (32.1551, 35.1091) centre (32.1551, 35.2678) ccw
  arc A1316 (33.7289, 35.8033) -> (33.5044, 36.0279) centre (33.6167, 35.9156) ccw
  line L300 (31.1961, 33.461) -> (31.5555, 33.3121)
  line L301 (34.9633, 32.6644) -> (35.9156, 33.6167)
  line L302 (29.5021, 35.3655) -> (29.651, 35.0061)
  arc A1317 (29.9261, 42.8978) -> (29.9261, 42.5803) centre (29.9261, 42.739) ccw
  arc A1318 (32.0808, 48.1801) -> (31.9593, 47.8868) centre (32.0201, 48.0335) ccw
  line L303 (24.0548, 46.7828) -> (23.7022, 46.4302)
  arc A1319 (34.4478, 47.9212) -> (34.6723, 48.1457) centre (34.5601, 48.0335) ccw
  arc A1320 (33.6167, 36.0743) -> (33.6167, 35.7568) centre (33.6167, 35.9156) ccw
  arc A1321 (31.5555, 33.4708) -> (31.5555, 33.1534) centre (31.5555, 33.3121) ccw
  arc A1322 (31.0332, 33.8483) -> (30.8087, 33.6238) centre (30.921, 33.7361) ccw
  arc A1323 (33.6167, 32.8231) -> (33.6167, 32.5057) centre (33.6167, 32.6644) ccw
  arc A1324 (29.7632, 35.1183) -> (29.5387, 34.8938) centre (29.651, 35.006) ccw
  arc A1325 (35.0756, 36.0279) -> (34.8511, 35.8033) centre (34.9634, 35.9156) ccw
  arc A1326 (23.3526, 45.4706) -> (23.6701, 45.4706) centre (23.5113, 45.4706) ccw
  arc A1327 (25.6724, 44.6298) -> (25.4478, 44.8544) centre (25.5601, 44.7421) ccw
  line L304 (25.5601, 44.7421) -> (31.9291, 44.7421)
  arc A1328 (25.0751, 47.1204) -> (24.9536, 46.827) centre (25.0144, 46.9737) ccw
  arc A1329 (29.5387, 42.5762) -> (29.7632, 42.3517) centre (29.6509, 42.4639) ccw
  line L305 (33.6167, 35.9156) -> (32.969, 35.2679)
  line L306 (32.969, 35.2679) -> (32.1551, 35.2679)
  arc A1330 (31.9291, 44.5834) -> (31.9291, 44.9008) centre (31.9291, 44.7421) ccw
  arc A1331 (29.5043, 34.9453) -> (29.7976, 35.0668) centre (29.651, 35.0061) ccw
  arc A1332 (29.6609, 42.1045) -> (29.3434, 42.1045) centre (29.5022, 42.1045) ccw
  arc A1333 (29.9261, 42.5803) -> (29.9261, 42.8978) centre (29.9261, 42.739) ccw
  line L307 (56.6547, 44.4709) -> (56.6547, 44.323)
  arc A1334 (58.8319, 46.0318) -> (58.7104, 45.7384) centre (58.7711, 45.8851) ccw
  arc A1335 (31.2568, 33.6076) -> (31.1353, 33.3143) centre (31.196, 33.461) ccw
  arc A1336 (59.2849, 45.8534) -> (59.2849, 46.1709) centre (59.2849, 46.0122) ccw
  arc A1337 (57.0701, 45.059) -> (56.7768, 45.1805) centre (56.9235, 45.1197) ccw
  arc A1338 (56.8135, 44.4709) -> (56.496, 44.4709) centre (56.6547, 44.4709) ccw
  line L308 (56.6547, 44.323) -> (54.5937, 44.323)
  arc A1339 (58.7711, 45.7263) -> (58.7711, 46.0438) centre (58.7711, 45.8851) ccw
  line L309 (57.42, 45.6163) -> (56.9235, 45.1198)
  line L310 (25.4752, 44.6572) -> (25.5601, 44.7421)
  arc A1340 (56.8112, 45.232) -> (57.0357, 45.0075) centre (56.9234, 45.1197) ccw
  arc A1341 (54.5937, 44.4817) -> (54.5937, 44.1642) centre (54.5937, 44.323) ccw
  arc A1342 (43.2923, 46.9893) -> (43.0677, 46.7648) centre (43.18, 46.8771) ccw
  arc A1343 (59.5777, 45.4586) -> (59.8023, 45.2341) centre (59.69, 45.3464) ccw
  arc A1344 (32.969, 33.1534) -> (32.969, 33.4708) centre (32.969, 33.3121) ccw
  line L311 (54.5937, 44.323) -> (54.5937, 44.6994)
  line L312 (59.2849, 46.0121) -> (59.8204, 45.4767)
  arc A1345 (32.0428, 35.1556) -> (32.2673, 35.3802) centre (32.1551, 35.2679) ccw
  line L313 (56.9235, 45.1198) -> (56.6547, 44.4709)
  arc A1346 (59.3972, 46.1244) -> (59.1727, 45.8998) centre (59.2849, 46.0121) ccw
  line L314 (59.8204, 45.4767) -> (59.69, 45.3463)
  arc A1347 (31.6166, 41.5049) -> (31.2991, 41.5049) centre (31.4579, 41.5049) ccw
  arc A1348 (56.496, 44.323) -> (56.8135, 44.323) centre (56.6547, 44.323) ccw
  arc A1349 (29.8138, 42.8513) -> (30.0383, 42.6268) centre (29.9261, 42.7391) ccw
  arc A1350 (29.6488, 35.4262) -> (29.3554, 35.3047) centre (29.5021, 35.3655) ccw
  arc A1351 (54.7524, 44.6994) -> (54.4349, 44.6994) centre (54.5937, 44.6994) ccw
  arc A1352 (56.6547, 44.1642) -> (56.6547, 44.4817) centre (56.6547, 44.323) ccw
  arc A1353 (33.5044, 32.5521) -> (33.7289, 32.7767) centre (33.6167, 32.6644) ccw
  line L315 (29.9261, 34.731) -> (30.921, 33.7361)
  arc A1354 (39.9847, 43.4743) -> (39.8632, 43.7676) centre (39.924, 43.621) ccw
  arc A1355 (31.2991, 35.9651) -> (31.6166, 35.9651) centre (31.4579, 35.9651) ccw
  arc A1356 (34.9633, 32.5057) -> (34.9633, 32.8231) centre (34.9633, 32.6644) ccw
  line L316 (59.42, 45.6163) -> (58.7711, 45.8851)
  line L317 (31.4579, 35.9651) -> (31.4579, 41.5049)
  arc A1357 (33.5373, 43.3598) -> (33.3128, 43.5844) centre (33.4251, 43.4721) ccw
  arc A1358 (29.9261, 34.5722) -> (29.9261, 34.8897) centre (29.9261, 34.7309) ccw
  arc A1359 (39.8117, 43.7332) -> (40.0362, 43.5087) centre (39.924, 43.621) ccw
  arc A1360 (59.9326, 45.3644) -> (59.7081, 45.5889) centre (59.8203, 45.4767) ccw
  arc A1361 (59.7081, 45.3644) -> (59.9326, 45.5889) centre (59.8203, 45.4767) ccw
  arc A1362 (58.0689, 46.0438) -> (58.0689, 45.7263) centre (58.0689, 45.8851) ccw
  arc A1363 (44.2555, 46.1709) -> (44.2555, 45.8534) centre (44.2555, 46.0122) ccw
  arc A1364 (54.4349, 44.323) -> (54.7524, 44.323) centre (54.5937, 44.323) ccw
  line L318 (31.9291, 44.7421) -> (29.9261, 42.739)
  line L319 (43.18, 46.877) -> (43.8961, 46.161)
  line L320 (32.969, 33.3121) -> (33.6167, 32.6644)
  arc A1365 (39.5645, 43.3134) -> (39.5645, 43.6309) centre (39.5645, 43.4721) ccw
  arc A1366 (56.508, 44.5317) -> (56.8014, 44.4102) centre (56.6547, 44.471) ccw
  arc A1367 (43.9568, 46.3076) -> (43.8353, 46.0143) centre (43.896, 46.161) ccw
  arc A1368 (59.5777, 45.2341) -> (59.8023, 45.4586) centre (59.69, 45.3464) ccw
  line L321 (40.199, 43.8961) -> (43.18, 46.877)
  arc A1369 (57.5323, 45.5041) -> (57.3078, 45.7286) centre (57.4201, 45.6164) ccw
  arc A1370 (44.1947, 45.8654) -> (44.3162, 46.1588) centre (44.2554, 46.0121) ccw
  line L322 (32.1551, 35.2679) -> (31.4579, 35.9651)
  arc A1371 (33.4251, 43.6309) -> (33.4251, 43.3134) centre (33.4251, 43.4721) ccw
  arc A1372 (40.3113, 43.7838) -> (40.0868, 44.0083) centre (40.199, 43.896) ccw
  arc A1373 (31.5702, 36.0773) -> (31.3456, 35.8528) centre (31.4579, 35.965) ccw
  line L323 (33.6167, 32.6644) -> (34.9633, 32.6644)
  line L324 (33.4251, 43.4721) -> (39.5645, 43.4721)
  arc A1374 (35.611, 39.2366) -> (35.611, 38.9191) centre (35.611, 39.0778) ccw
  arc A1375 (32.5057, 37.4267) -> (32.8231, 37.4267) centre (32.6644, 37.4267) ccw
  line L325 (42.351, 45.0039) -> (40.7429, 43.3959)
  arc A1376 (34.9633, 36.3157) -> (34.9633, 36.6332) centre (34.9633, 36.4745) ccw
  arc A1377 (39.2664, 41.6948) -> (39.0418, 41.9193) centre (39.1541, 41.807) ccw
  line L326 (39.1541, 42.5255) -> (39.1541, 41.8071)
  arc A1378 (43.2923, 46.7648) -> (43.0677, 46.9893) centre (43.18, 46.877) ccw
  line L327 (52.6298, 45.5128) -> (52.5449, 45.4279)
  line L328 (33.6167, 36.4744) -> (34.9633, 36.4744)
  line L329 (58.7711, 45.8851) -> (58.0689, 45.8851)
  arc A1379 (53.0906, 45.8624) -> (53.0906, 45.5449) centre (53.0906, 45.7036) ccw
  arc A1380 (43.7838, 46.0487) -> (44.0083, 46.2732) centre (43.896, 46.1609) ccw
  line L330 (34.9633, 39.7256) -> (33.6167, 39.7256)
  arc A1381 (40.0245, 43.5546) -> (40.0245, 43.2371) centre (40.0245, 43.3959) ccw
  line L331 (35.611, 39.0779) -> (34.9633, 39.7256)
  arc A1382 (33.7289, 39.6133) -> (33.5044, 39.8379) centre (33.6167, 39.7256) ccw
  arc A1383 (52.4326, 45.5402) -> (52.6572, 45.3156) centre (52.5449, 45.4279) ccw
  arc A1384 (42.9855, 45.5866) -> (42.9855, 45.2691) centre (42.9855, 45.4278) ccw
  arc A1385 (40.0868, 44.0083) -> (40.3113, 43.7838) centre (40.199, 43.896) ccw
  arc A1386 (54.1624, 45.6251) -> (53.9379, 45.4006) centre (54.0502, 45.5129) ccw
  arc A1387 (42.2387, 45.1162) -> (42.4632, 44.8917) centre (42.351, 45.004) ccw
  arc A1388 (42.7383, 45.1668) -> (42.5138, 45.3913) centre (42.6261, 45.2791) ccw
  line L332 (31.4579, 41.5049) -> (33.4251, 43.4721)
  arc A1389 (59.3592, 45.4697) -> (59.4807, 45.763) centre (59.42, 45.6163) ccw
  line L333 (44.2555, 46.0121) -> (59.2849, 46.0121)
  line L334 (39.5645, 43.4721) -> (39.9239, 43.621)
  arc A1390 (38.9954, 41.8071) -> (39.3128, 41.8071) centre (39.1541, 41.8071) ccw
  line L335 (32.6644, 37.4267) -> (33.6167, 36.4744)
  line L336 (54.5937, 44.6994) -> (54.4028, 45.1602)
  arc A1391 (36.3127, 39.1902) -> (36.5372, 38.9656) centre (36.425, 39.0779) ccw
  arc A1392 (33.6167, 39.8843) -> (33.6167, 39.5668) centre (33.6167, 39.7256) ccw
  arc A1393 (34.9633, 39.5668) -> (34.9633, 39.8843) centre (34.9633, 39.7256) ccw
  arc A1394 (42.5097, 45.0039) -> (42.1922, 45.0039) centre (42.351, 45.0039) ccw
  arc A1395 (33.5044, 36.3621) -> (33.7289, 36.5867) centre (33.6167, 36.4744) ccw
  line L337 (58.0689, 45.8851) -> (57.42, 45.6163)
  arc A1396 (52.5691, 45.6595) -> (52.6906, 45.3662) centre (52.6299, 45.5129) ccw
  arc A1397 (31.3456, 41.6172) -> (31.5701, 41.3927) centre (31.4579, 41.5049) ccw
  arc A1398 (59.5322, 45.7286) -> (59.3077, 45.5041) centre (59.4199, 45.6164) ccw
  arc A1399 (58.1296, 45.7384) -> (58.0081, 46.0318) centre (58.0688, 45.8851) ccw
  line L338 (53.5894, 45.7037) -> (53.0906, 45.7037)
  arc A1400 (53.1514, 45.557) -> (53.0299, 45.8504) centre (53.0907, 45.7037) ccw
  arc A1401 (40.6307, 43.5082) -> (40.8552, 43.2836) centre (40.743, 43.3959) ccw
  line L339 (40.0245, 43.3959) -> (39.1541, 42.5255)
  arc A1402 (53.5894, 45.5449) -> (53.5894, 45.8624) centre (53.5894, 45.7036) ccw
  line L340 (52.5449, 45.4279) -> (42.9855, 45.4279)
  line L341 (43.8961, 46.161) -> (44.2555, 46.0121)
  arc A1403 (43.0462, 45.2812) -> (42.9247, 45.5746) centre (42.9855, 45.4279) ccw
  line L342 (40.7429, 43.3959) -> (40.0245, 43.3959)
  arc A1404 (32.7767, 37.5389) -> (32.5521, 37.3144) centre (32.6644, 37.4267) ccw
  arc A1405 (54.2906, 45.0479) -> (54.5151, 45.2724) centre (54.4028, 45.1601) ccw
  arc A1406 (57.3593, 45.763) -> (57.4808, 45.4697) centre (57.4201, 45.6163) ccw
  line L343 (59.69, 45.3463) -> (59.42, 45.6163)
  line L344 (39.9239, 43.621) -> (40.199, 43.8961)
  arc A1407 (32.8231, 38.7733) -> (32.5057, 38.7733) centre (32.6644, 38.7733) ccw
  line L345 (36.4249, 39.0779) -> (35.611, 39.0779)
  arc A1408 (54.5495, 45.2209) -> (54.2562, 45.0994) centre (54.4029, 45.1602) ccw
  arc A1409 (35.4988, 38.9656) -> (35.7233, 39.1902) centre (35.6111, 39.0779) ccw
  arc A1410 (32.969, 35.1091) -> (32.969, 35.4266) centre (32.969, 35.2678) ccw
  arc A1411 (53.9894, 45.3662) -> (54.1109, 45.6595) centre (54.0502, 45.5129) ccw
  arc A1412 (39.5038, 43.6188) -> (39.6253, 43.3254) centre (39.5645, 43.4721) ccw
  arc A1413 (54.447, 44.6386) -> (54.7404, 44.7601) centre (54.5937, 44.6993) ccw
  line L346 (54.0502, 45.5128) -> (53.5894, 45.7037)
  arc A1414 (39.3128, 42.5255) -> (38.9954, 42.5255) centre (39.1541, 42.5255) ccw
  arc A1415 (42.2846, 42.0129) -> (41.9671, 42.0129) centre (42.1258, 42.0129) ccw
  line L347 (50.7457, 43.4721) -> (50.6695, 43.3959)
  line L348 (39.1541, 38.7155) -> (39.1541, 37.4845)
  arc A1416 (50.2968, 43.2836) -> (50.0723, 43.5082) centre (50.1846, 43.3959) ccw
  arc A1417 (49.0566, 41.6242) -> (49.0566, 41.9417) centre (49.0566, 41.7829) ccw
  arc A1418 (40.1368, 43.2836) -> (39.9123, 43.5082) centre (40.0246, 43.3959) ccw
  arc A1419 (49.4264, 41.9283) -> (49.2018, 42.1528) centre (49.3141, 42.0406) ccw
  line L349 (49.3141, 42.0405) -> (49.0566, 41.783)
  arc A1420 (50.1845, 43.5546) -> (50.1845, 43.2371) centre (50.1845, 43.3959) ccw
  line L350 (34.9633, 36.4744) -> (35.611, 37.1221)
  line L351 (42.6261, 45.279) -> (42.351, 45.0039)
  arc A1421 (39.0418, 38.8277) -> (39.2664, 38.6032) centre (39.1541, 38.7155) ccw
  arc A1422 (40.1368, 39.4736) -> (39.9123, 39.6982) centre (40.0246, 39.5859) ccw
  arc A1423 (36.9638, 37.2688) -> (37.0853, 36.9754) centre (37.0245, 37.1221) ccw
  line L352 (40.5371, 40.4241) -> (41.2555, 40.4241)
  arc A1424 (35.7233, 37.0098) -> (35.4988, 37.2344) centre (35.611, 37.1221) ccw
  line L353 (43.5851, 43.4721) -> (50.7457, 43.4721)
  line L354 (32.6644, 38.7733) -> (32.6644, 37.4267)
  line L355 (33.6167, 39.7256) -> (32.6644, 38.7733)
  arc A1425 (40.7429, 43.2371) -> (40.7429, 43.5546) centre (40.7429, 43.3959) ccw
  arc A1426 (32.5521, 38.8856) -> (32.7767, 38.6611) centre (32.6644, 38.7734) ccw
  line L356 (35.611, 37.1221) -> (37.0245, 37.1221)
  line L357 (49.3141, 42.5255) -> (49.3141, 42.0405)
  arc A1427 (42.4632, 44.8917) -> (42.2387, 45.1162) centre (42.351, 45.004) ccw
  line L358 (42.211, 41.2875) -> (40.5095, 39.5859)
  arc A1428 (42.6448, 41.4967) -> (42.4203, 41.7212) centre (42.5325, 41.609) ccw
  arc A1429 (42.5653, 45.4257) -> (42.6868, 45.1324) centre (42.6261, 45.2791) ccw
  line L359 (40.0245, 39.5859) -> (39.1541, 38.7155)
  arc A1430 (35.0756, 39.8379) -> (34.8511, 39.6133) centre (34.9634, 39.7256) ccw
  arc A1431 (40.5371, 40.5829) -> (40.5371, 40.2654) centre (40.5371, 40.4241) ccw
  arc A1432 (43.6973, 43.3598) -> (43.4728, 43.5844) centre (43.585, 43.4721) ccw
  arc A1433 (53.6501, 45.8504) -> (53.5286, 45.557) centre (53.5894, 45.7037) ccw
  line L360 (37.3839, 37.271) -> (40.5371, 40.4241)
  arc A1434 (50.6695, 43.2371) -> (50.6695, 43.5546) centre (50.6695, 43.3959) ccw
  arc A1435 (42.0136, 42.1252) -> (42.2382, 41.9007) centre (42.1259, 42.013) ccw
  arc A1436 (41.9671, 41.2945) -> (42.2846, 41.2945) centre (42.1258, 41.2945) ccw
  line L361 (40.5095, 39.5859) -> (40.0245, 39.5859)
  arc A1437 (37.2717, 37.3832) -> (37.4962, 37.1587) centre (37.384, 37.2709) ccw
  arc A1438 (50.5572, 43.5082) -> (50.7817, 43.2836) centre (50.6694, 43.3959) ccw
  arc A1439 (40.3972, 39.6982) -> (40.6217, 39.4736) centre (40.5094, 39.5859) ccw
  arc A1440 (40.5095, 39.4271) -> (40.5095, 39.7446) centre (40.5095, 39.5859) ccw
  arc A1441 (42.4718, 41.7557) -> (42.5933, 41.4623) centre (42.5326, 41.609) ccw
  arc A1442 (39.3128, 38.7155) -> (38.9954, 38.7155) centre (39.1541, 38.7155) ccw
  arc A1443 (39.0418, 42.6377) -> (39.2664, 42.4132) centre (39.1541, 42.5255) ccw
  line L362 (53.0906, 45.7037) -> (52.6298, 45.5128)
  line L363 (39.1541, 41.8071) -> (36.4249, 39.0779)
  arc A1444 (42.3233, 41.1752) -> (42.0988, 41.3997) centre (42.2111, 41.2875) ccw
  arc A1445 (37.4447, 37.1243) -> (37.3232, 37.4176) centre (37.3839, 37.2709) ccw
  arc A1446 (52.7421, 45.4006) -> (52.5176, 45.6251) centre (52.6299, 45.5129) ccw
  line L364 (42.9855, 45.4279) -> (42.6261, 45.279)
  line L365 (37.0245, 37.1221) -> (37.3839, 37.271)
  arc A1447 (49.4729, 42.5255) -> (49.1554, 42.5255) centre (49.3142, 42.5255) ccw
  line L366 (54.4028, 45.1602) -> (54.0502, 45.5128)
  arc A1448 (36.4249, 38.9191) -> (36.4249, 39.2366) centre (36.4249, 39.0778) ccw
  arc A1449 (52.5449, 45.2691) -> (52.5449, 45.5866) centre (52.5449, 45.4278) ccw
  arc A1450 (40.6493, 40.3118) -> (40.4248, 40.5364) centre (40.537, 40.4241) ccw
  arc A1451 (38.9954, 37.4845) -> (39.3128, 37.4845) centre (39.1541, 37.4845) ccw
  arc A1452 (42.1922, 45.0039) -> (42.5097, 45.0039) centre (42.351, 45.0039) ccw
  arc A1453 (40.0245, 39.7446) -> (40.0245, 39.4271) centre (40.0245, 39.5859) ccw
  arc A1454 (50.8579, 43.3598) -> (50.6334, 43.5844) centre (50.7457, 43.4721) ccw
  arc A1455 (42.2382, 41.1823) -> (42.0136, 41.4068) centre (42.1259, 41.2945) ccw
  arc A1456 (41.1432, 40.5364) -> (41.3677, 40.3118) centre (41.2554, 40.4241) ccw
  line L367 (42.5325, 41.609) -> (42.211, 41.2875)
  arc A1457 (43.7657, 39.3847) -> (43.5412, 39.6093) centre (43.6535, 39.497) ccw
  line L368 (57.42, 40.7437) -> (58.0689, 40.4749)
  arc A1458 (51.0428, 40.3118) -> (50.8183, 40.5364) centre (50.9306, 40.4241) ccw
  arc A1459 (50.7457, 43.3134) -> (50.7457, 43.6309) centre (50.7457, 43.4721) ccw
  arc A1460 (58.7104, 40.6216) -> (58.8319, 40.3282) centre (58.7711, 40.4749) ccw